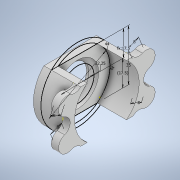
# Autodesk Inventor part: shaft holder
Saved by Autodesk Inventor 2020.3 (Build 243373000, 373)
## iProperties
Created: 2020-08-09
Part Number: shaft holder
Material: Generic
Document SubType Name: Modeling
Designer: joesp
Density: 1 g/cm^3
Appearance: Default
Author: joesp
Autodesk Inventor part; units mm, degrees
ref_plane "YZ Plane" through (0, 0, 0) normal (1, 0, 0) x (0, 1, 0)
ref_plane "XZ Plane" through (0, 0, 0) normal (0, 1, 0) x (-1, 0, 0)
ref_plane "XY Plane" through (0, 0, 0) normal (0, 0, 1) x (1, 0, 0)
sketch "Sketch1" plane through (0, 0, 0) normal (1, 0, 0) x (0, 1, 0)
  circle A0 centre (0, 0) radius 11.125
  line L0 (17.5, 17.8536) -> (17.5, -17.8536)
  line L1 (-17.5, 17.8536) -> (-17.5, -17.8536)
  circle A1 centre (0, 0) radius 25
  circle A2 centre (0, 0) radius 22
  point P0 (-17.5, -13.3323)
  point P1 (17.5, -13.3323)
  point P2 (17.5, 13.3323)
  point P3 (-17.5, 13.3323)
  dimension "d0" = 22.25
  dimension "d1" = 44
  dimension "d2" = 3
  dimension "d3" = 35
  dimension "d4" = 17.5
  dimension "d5" = 17.5
  constraints: 4 end point, 4 point on circle, 3 centre point, 3 coincident, 2 vertical
  measures "d0" diameter of A0
  measures "d1" diameter of A2
  measures "d2" radial gap between concentric circles of A1 A2
  measures "d3" distance between parallel lines of L1 L0
  measures "d4" distance from line of point (0, 0) L0
  measures "d5" distance from line of point (0, 0) L1
extrude "Extrusion1" add sketch "Sketch1" against normal blind 5 contours L0 A2 L1
sketch "Sketch2" plane through (0, 0, 0) normal (0, 1, 0) x (-1, 0, 0)
  circle A0 centre (1, -12.125) radius 2.5
  line L0 (0, -11.125) -> (0, 11.125) projected
  line L1 (0, -13.3323) -> (5, -13.3323) projected
  line L2 (10.1054, 0) -> (-6.8503, 0) construction
  point P0 (0, 0)
  dimension "d8" = 5
  dimension "d9" = 1
  dimension "d11" = 1
  constraints: 2 end point, 1 centre point, 1 coincident, 1 horizontal
  measures "d8" diameter of A0
  measures "d9" distance from line of L0 A0.centre
  measures "d11" horizontal distance of point (0, -11.125) A0.centre
revolve "Revolution1" cut sketch "Sketch2" angle 360 about axis through (-10.1054, 0, 0) along (1, 0, 0)
extrude "Extrusion2" add sketch "Sketch1" along normal blind 20 and the other way blind 5 contours L0 A2 L1 A1 | L0 A1 L1 A2
sketch "Sketch3" plane through (20, 0, 0) normal (1, 0, 0) x (0, 0, -1)
  line L0 (-13.3323, 17.5) -> (-17.8536, 17.5) projected
  arc A0 (-24.2536, 16.374) -> (-17.8536, 17.5) centre (-21.8402, 21.4076) ccw
  arc A1 (-24.2536, 16.374) -> (-28.7823, 5.2842) centre (-26.8477, 10.9637) ccw
  arc A2 (-17.8536, 17.5) -> (-17.8536, -17.5) centre (0, 0) ccw projected
  arc A3 (-25, 0) -> (-28.7823, 5.2842) centre (-30.5823, 0) ccw
  arc A4 (-28.7823, -5.2842) -> (-25, 0) centre (-30.5823, 0) ccw
  arc A5 (-28.7823, -5.2842) -> (-24.2536, -16.374) centre (-26.8477, -10.9637) ccw
  arc A6 (-17.8536, -17.5) -> (-24.2536, -16.374) centre (-21.8402, -21.4076) ccw
  arc A7 (-17.8536, 17.5) -> (-17.8536, -17.5) centre (0, 0) ccw projected
  line L1 (-17.8536, 17.5) -> (17.8536, 17.5) projected
  arc A8 (17.8536, 17.5) -> (24.2536, 16.374) centre (21.8402, 21.4076) ccw
  arc A9 (28.7823, 5.2842) -> (24.2536, 16.374) centre (26.8477, 10.9637) ccw
  arc A10 (28.7823, 5.2842) -> (25, 0) centre (30.5823, 0) ccw
  line L2 (17.8536, -17.5) -> (-17.8536, -17.5) projected
  arc A11 (24.2536, -16.374) -> (17.8536, -17.5) centre (21.8402, -21.4076) ccw
  arc A12 (24.2536, -16.374) -> (28.7823, -5.2842) centre (26.8477, -10.9637) ccw
  arc A13 (25, 0) -> (28.7823, -5.2842) centre (30.5823, 0) ccw
  arc A14 (17.8536, -17.5) -> (17.8536, 17.5) centre (0, 0) ccw projected
  circle A15 centre (-26.8477, -10.9637) radius 4 construction
  circle A16 centre (-26.8477, 10.9637) radius 4 construction
  circle A17 centre (26.8477, 10.9637) radius 4 construction
  circle A18 centre (26.8477, -10.9637) radius 4 construction
  dimension "d17" = 6
  dimension "d18" = 6
  dimension "d19" = 6
  dimension "d20" = 6
  dimension "d21" = 8
  dimension "d22" = 8
  dimension "d23" = 8
  dimension "d24" = 8
  constraints: 27 point on circle, 19 tangent, 16 centre point, 4 coincident, 2 equal radius, 2 horizontal alignment, 2 vertical alignment
  measures "d17" radius of A5
  measures "d18" radius of A12
  measures "d19" radius of A1
  measures "d20" radius of A9
  measures "d21" diameter of A15
  measures "d22" diameter of A16
  measures "d23" diameter of A17
  measures "d24" diameter of A18
extrude "Extrusion3" add sketch "Sketch3" against normal blind 5 contours A2 A3 A1 A0 | A8 A9 A10 A14 | A2 A6 A5 A4 | A13 A12 A11 A14
sketch "Sketch4" plane through (15, 0, 0) normal (-1, 0, 0) x (0, 0, 1)
  line L0 (22.5385, -11.0612) -> (24.1834, -6.7452)
  line L1 (24.1834, -6.7452) -> (28.7436, -6.0118)
  line L2 (28.7436, -6.0118) -> (31.6589, -9.5943)
  line L3 (31.6589, -9.5943) -> (30.014, -13.9102)
  line L4 (30.014, -13.9102) -> (25.4538, -14.6437)
  line L5 (25.4538, -14.6437) -> (22.5385, -11.0612)
  line L6 (24.8797, 15.5992) -> (29.4644, 15.0393)
  line L7 (29.4644, 15.0393) -> (31.2719, 10.7889)
  line L8 (31.2719, 10.7889) -> (28.4947, 7.0983)
  line L9 (28.4947, 7.0983) -> (23.9099, 7.6582)
  line L10 (23.9099, 7.6582) -> (22.1024, 11.9086)
  line L11 (22.1024, 11.9086) -> (24.8797, 15.5992)
  line L12 (-25.1584, -15.1456) -> (-29.7322, -14.5027)
  line L13 (-29.7322, -14.5027) -> (-31.4624, -10.2202)
  line L14 (-31.4624, -10.2202) -> (-28.6187, -6.5806)
  line L15 (-28.6187, -6.5806) -> (-24.0448, -7.2235)
  line L16 (-24.0448, -7.2235) -> (-22.3147, -11.506)
  line L17 (-22.3147, -11.506) -> (-25.1584, -15.1456)
  line L18 (-29.7136, 14.5408) -> (-25.1389, 15.1779)
  line L19 (-25.1389, 15.1779) -> (-22.2999, 11.5346)
  line L20 (-22.2999, 11.5346) -> (-24.0356, 7.2543)
  line L21 (-24.0356, 7.2543) -> (-28.6102, 6.6173)
  line L22 (-28.6102, 6.6173) -> (-31.4492, 10.2606)
  line L23 (-31.4492, 10.2606) -> (-29.7136, 14.5408)
  arc A0 (17.8536, -17.5) -> (17.8536, 17.5) centre (0, 0) ccw projected
  arc A1 (-17.8536, 17.5) -> (-17.8536, -17.5) centre (0, 0) ccw projected
  point P0 (27.0987, -10.3277)
  point P1 (26.6872, 11.3487)
  point P2 (-26.8885, -10.8631)
  point P3 (-26.8746, 10.8976)
  point P4 (23.0062, 9.7834)
  point P5 (23.3609, -8.9032)
  point P6 (-23.1798, -9.3647)
  point P7 (-23.1677, 9.3945)
  dimension "d27" = 8
  dimension "d30" = 8
  dimension "d31" = 8
  dimension "d32" = 8
  constraints: 48 end point, 4 midpoint, 4 point on circle, 4 tangent, 52 other
  measures "d27" distance between parallel lines of L10 L7
  measures "d30" distance between parallel lines of L0 L3
  measures "d31" distance between parallel lines of L13 L16
  measures "d32" distance between parallel lines of L23 L20
equation "\"d4\" = d5"
equation "\"d18\" = d17"
equation "\"d19\" = d17"
equation "\"d20\" = d17"
equation "\"d22\" = d21"
equation "\"d23\" = d21"
equation "\"d24\" = d21"
body "Solid1"
